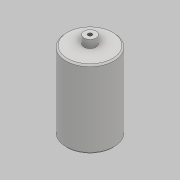
# Autodesk Inventor part: exercise3-11
Saved by Autodesk Inventor 2018 (Build 220112000, 112)
## iProperties
Created: 2020-09-23
Part Number: exercise3-11
Material: 一般
Document SubType Name: Modeling
Designer: 王鼎鈞
Density: 1 g/cm^3
Appearance: 預設
Author: 王鼎鈞
Autodesk Inventor part; units mm, degrees
ref_plane "YZ Plane" through (0, 0, 0) normal (1, 0, 0) x (0, 1, 0)
ref_plane "XZ Plane" through (0, 0, 0) normal (0, 1, 0) x (-1, 0, 0)
ref_plane "XY Plane" through (0, 0, 0) normal (0, 0, 1) x (1, 0, 0)
sketch "草圖1" plane through (0, 0, 0) normal (1, 0, 0) x (0, 1, 0)
  line L0 (-26.8, 0) -> (62.8, 0) projected
  line L1 (0, -120) -> (0, 20) projected
  line L2 (-14, -100) -> (14, -100)
  line L3 (0, -100) -> (12.5, -100)
  line L4 (12.5, -100) -> (12.5, -83.5)
  line L5 (12.5, -83.5) -> (0, -83.5)
  line L6 (0, -83.5) -> (0, -100)
  line L7 (12.5, -83.5) -> (50, -80.2192)
  line L8 (12.5, -83.5) -> (37.1972, -83.5) construction
  line L9 (50, -80.2192) -> (50, 0)
  line L10 (50, 0) -> (0, 0)
  line L11 (0, 0) -> (0, -83.5)
  dimension "d0" = 100
  dimension "d1" = 12.5
  dimension "d2" = 16.5
  dimension "d3" = 0
  dimension "d4" = 5
  dimension "d5" = 50
  constraints: 20 end point, 4 parallel, 2 horizontal, 1 collinear, 1 midpoint, 1 perpendicular, 1 point on line
  measures "d0" distance between parallel lines of L0 L2
  measures "d1" distance of L5.end L4.end
  measures "d2" distance of L4.end L3.end
  measures "d3" distance between parallel lines of L1 L6
  measures "d4" angle of L8 L7
  measures "d5" distance between parallel lines of L1 L9
revolve "迴轉1" add sketch "草圖1" angle 360 about axis through (0, 0, 0) along (0, 0, -1)
mirror "鏡射1" about plane through (0, 50, 0) normal (0, 0, 1) of "迴轉1"
chamfer "倒角1" distance 3 angle 45 2 edges at (0, -50, 80.2192) (0, -50, -80.2192)
hole "孔1" at (0, 0, 100) direction (0, 0, -1) diameter 8.376 depth 59 tip angle 118 thread size "M10x1.5" class "6H" standard "ISO Metric profile"
ref_plane "工作平面1" through (0, 0, 0) normal (0, 0, 1) x (1, 0, 0)
ref_plane "工作平面2" through (0, 0, 0) normal (0, 0, -1) x (-1, 0, 0)
mirror "鏡射2" about plane through (0, 0, 0) normal (0, 0, 1) of "孔1"
